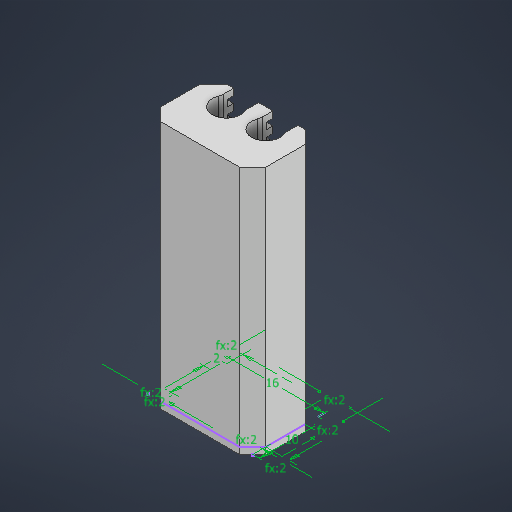
# Autodesk Inventor part: Test
Saved by Autodesk Inventor 2026.2 (Build 302298000, 298)
## iProperties
Created: 2026-01-26
Part Number: Test
Material: Generic
Document SubType Name: Modeling
Designer: Cobble
Density: 1 g/cm^3
Appearance: Default
Author: Cobble
Autodesk Inventor part; units mm, degrees
ref_plane "YZ Plane" through (0, 0, 0) normal (1, 0, 0) x (0, 1, 0)
ref_plane "XZ Plane" through (0, 0, 0) normal (0, 1, 0) x (-1, 0, 0)
ref_plane "XY Plane" through (0, 0, 0) normal (0, 0, 1) x (1, 0, 0)
sketch "Sketch1" plane through (0, 0, 0) normal (0, 0, 1) x (1, 0, 0)
  line L0 (-2, -4) -> (10, -4)
  line L1 (12, -2) -> (12, 4)
  line L2 (10, 6) -> (-2, 6)
  line L3 (-4, 4) -> (-4, -2)
  line L4 (-4, 7.1505) -> (-4, 6)
  line L5 (12, 6) -> (12, 7.1505)
  line L6 (-4, 4) -> (-2, 6)
  line L7 (10, 6) -> (12, 4)
  line L8 (12, -2) -> (10, -4)
  line L9 (-2, -4) -> (-4, -2)
  line L10 (-3, 5) -> (11, 5)
  point P0 (-4, -4)
  point P1 (12, -4)
  dimension "d12" = 16
  dimension "d13" = 10
  dimension "d18" = 2
  dimension "d19" = 2
  dimension "d20" = 2
  dimension "d21" = 2
  dimension "d22" = 2
  dimension "d23" = 2
  dimension "d24" = 2
  dimension "d25" = 2
  constraints: 22 end point, 8 point on line, 2 midpoint, 2 parallel, 2 perpendicular, 1 horizontal, 1 vertical
  measures "d12" distance of L4.end L5.start
  measures "d13" distance of L5.start point (12, -4)
  measures "d18" distance of L3.start L4.end
  measures "d19" distance of L2.end L4.end
  measures "d20" distance of L2.start L5.start
  measures "d21" distance of L1.end L5.start
  measures "d22" distance of L1.start point (12, -4)
  measures "d23" distance of L0.end point (12, -4)
  measures "d24" distance of L0.start point (-4, -4)
  measures "d25" distance of L3.end point (-4, -4)
extrude "Extrusion1" add sketch "Sketch1" along normal blind 1
extrude "Extrusion2" add sketch "Sketch1" against normal blind 1 contours L9 L3 L6 L10 L7 L1 L8 L0
pattern_linear "Rectangular Pattern1" count 19 spacing 2 along (0, 0, 1) of "Extrusion1", "Extrusion2"
sketch "Sketch2" plane through (-2, -4, 37) normal (0, 0, 1) x (1, 0, 0)
  line L0 (0, 10) -> (-2, 8) projected
  line L1 (-2, 8) -> (-2, 2) projected
  line L2 (-2, 2) -> (0, 0) projected
  line L3 (0, 0) -> (12, 0) projected
  line L4 (12, 0) -> (14, 2) projected
  line L5 (14, 2) -> (14, 8) projected
  line L6 (14, 8) -> (12, 10) projected
  line L7 (12, 10) -> (0, 10) projected
  line L8 (0, 10) -> (12, 10)
  line L9 (6, 10) -> (8, 10)
  line L10 (6, 10) -> (0, 10)
  line L11 (3, 10) -> (3, 7)
  line L12 (3, 10) -> (6, 10) construction
  circle A0 centre (3, 7) radius 2.15
  line L13 (6, 10) -> (6, 0)
  line L14 (3, 10) -> (1.1, 10)
  line L15 (12, 10) -> (0, 10) projected
  line L16 (1.1, 10) -> (1.1, 8.0062)
  line L17 (1.1, 10) -> (4.9, 10)
  line L18 (4.9, 10) -> (4.9, 8.0062)
  line L19 (9, 10) -> (9, 7)
  circle A1 centre (9, 7) radius 2.15
  line L20 (10.9, 10) -> (10.9, 8.0062)
  line L21 (7.1, 10) -> (7.1, 8.0062)
  point P0 (2, 4)
  point P1 (9, 9.15)
  point P2 (4.9, 10)
  dimension "d39" = 3
  dimension "d40" = 90
  dimension "d41" = 4.3
  dimension "d42" = 1.9
  dimension "d43" = 3.8
  constraints: 26 end point, 7 symmetric about line, 4 point on circle, 3 midpoint, 3 perpendicular, 3 point on line, 2 centre point, 2 coincident, 2 horizontal, 1 collinear, 1 vertical, 1 other
  measures "d39" distance of L11.start L11.end
  measures "d40" angle of L11 L12
  measures "d41" diameter of A0
  measures "d42" distance of L11.start L14.end
  measures "d43" distance of L14.end L17.end
extrude "Extrusion3" cut sketch "Sketch2" against normal through all contours L7 L11 A0 L16 | L7 L18 A0 L11 | A0 | L7 L19 A1 L21 | A1 | L7 L20 A1 L19
fillet "Fillet1" radius 2 4 edges at (-0.9, 4.0062, 18) (2.9, 4.0062, 18) (8.9, 4.0062, 18) (5.1, 4.0062, 18)
equation "\"d19\" = d18"
equation "\"d20\" = d18"
equation "\"d21\" = d20"
equation "\"d22\" = d18"
equation "\"d23\" = d22"
equation "\"d24\" = d18"
equation "\"d25\" = d24"
equation "\"d41\" = Schlauch"
equation "\"Schlauch\" = 4.3"
body "Solid1"
